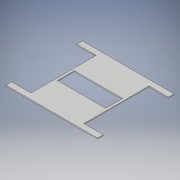
# Autodesk Inventor part: pcb_bottom
Saved by Autodesk Inventor 2019 (Build 230136000, 136)
## iProperties
Created: 2019-01-31
Part Number: pcb_bottom
Material: Ogólny
Document SubType Name: Modeling
Designer: atmat
Density: 1 g/cm^3
Appearance: Domyślna
Author: atmat
Autodesk Inventor part; units mm, degrees
ref_plane "YZ Plane" through (0, 0, 0) normal (1, 0, 0) x (0, 1, 0)
ref_plane "XZ Plane" through (0, 0, 0) normal (0, 1, 0) x (-1, 0, 0)
ref_plane "XY Plane" through (0, 0, 0) normal (0, 0, 1) x (1, 0, 0)
sketch "Szkic1" plane through (0, 0, 0) normal (0, 1, 0) x (-1, 0, 0)
  line L0 (-28, -40.5) -> (28, -40.5)
  line L1 (28, -40.5) -> (28, 40.5)
  line L2 (28, 40.5) -> (-28, 40.5)
  line L3 (-28, 40.5) -> (-28, -40.5)
  point P0 (0, 0)
  dimension "d0" = 81
  dimension "d1" = 56
  dimension "d2" = 28
  dimension "d3" = 40.5
  constraints: 8 end point, 2 parallel, 1 horizontal, 1 perpendicular
  measures "d0" distance of L0.end L1.end
  measures "d1" distance of L1.end L2.end
  measures "d2" distance from line of point (0, 0) L1
  measures "d3" distance from line of L2 point (0, 0)
extrude "Wyciągnięcie proste1" add sketch "Szkic1" along normal blind 1
sketch "Szkic2" plane through (0, 1, 0) normal (0, 1, 0) x (1, 0, 0)
  line L0 (-25.5, 9) -> (25.5, 9)
  line L1 (25.5, 9) -> (25.5, -9)
  line L2 (25.5, -9) -> (-25.5, -9)
  line L3 (-25.5, -9) -> (-25.5, 9)
  point P0 (0, 0)
  dimension "d6" = 18
  dimension "d7" = 9
  dimension "d8" = 51
  dimension "d9" = 25.5
  constraints: 8 end point, 2 parallel, 1 horizontal, 1 perpendicular
  measures "d6" distance of L0.end L1.end
  measures "d7" distance from line of point (0, 0) L0
  measures "d8" distance between parallel lines of L1 L3
  measures "d9" distance from line of point (0, 0) L3
extrude "Wyciągnięcie proste2" cut sketch "Szkic2" against normal blind 1
sketch "Szkic3" plane through (0, 1, 0) normal (0, 1, 0) x (1, 0, 0)
  line L0 (-48.5, -34.5) -> (48.5, -34.5)
  line L1 (48.5, -34.5) -> (48.5, -40.5)
  line L2 (48.5, -40.5) -> (-48.5, -40.5)
  line L3 (-48.5, -40.5) -> (-48.5, -34.5)
  line L4 (-28, -40.5) -> (28, -40.5) projected
  line L5 (25.5, -9) -> (-25.5, -9) projected
  line L6 (-48.5, 40.5) -> (48.5, 40.5)
  line L7 (48.5, 40.5) -> (48.5, 34.5)
  line L8 (48.5, 34.5) -> (-48.5, 34.5)
  line L9 (-48.5, 34.5) -> (-48.5, 40.5)
  line L10 (28, 40.5) -> (-28, 40.5) projected
  point P0 (0, 0)
  point P1 (28, -9.365)
  point P2 (-28, -9.365)
  point P3 (-25.5, -9)
  dimension "d12" = 97
  dimension "d13" = 6
  dimension "d15" = 48.5
  dimension "d17" = 0
  dimension "d20" = 6
  dimension "d21" = 0
  dimension "d22" = 97
  dimension "d23" = 0
  constraints: 16 end point, 4 parallel, 2 horizontal, 2 perpendicular, 1 other
  measures "d12" distance of L1.end L2.end
  measures "d13" distance of L2.end L0.start
  measures "d15" distance from line of point (0, 0) L3
  measures "d17" distance between parallel lines of L2 L4
  measures "d20" distance of L8.end L6.start
  measures "d21" distance between parallel lines of L10 L6
  measures "d22" distance of L7.end L8.end
  measures "d23" distance between parallel lines of L3 L9
extrude "Wyciągnięcie proste4" add sketch "Szkic3" against normal blind 1
